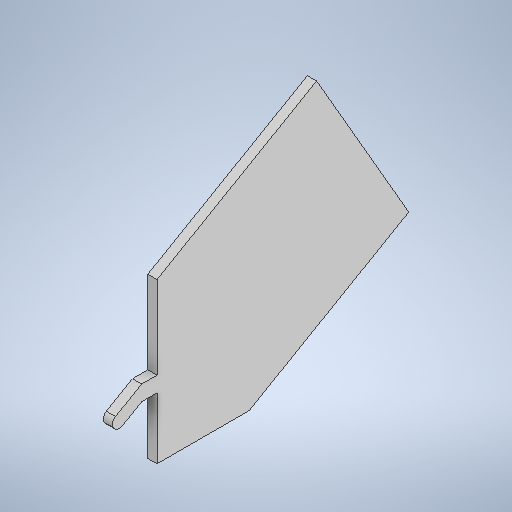
# Autodesk Inventor part: autour hélice
Saved by Autodesk Inventor 2026.2 (Build 302298010, 298A)
## iProperties
Created: 2026-04-02
Part Number: autour hélice
Material: Générique
Document SubType Name: Modeling
Designer: Genon
Density: 1 g/cm^3
Appearance: Par défaut
Author: Genon
Autodesk Inventor part; units mm, degrees
ref_plane "YZ Plane" through (0, 0, 0) normal (1, 0, 0) x (0, 1, 0)
ref_plane "XZ Plane" through (0, 0, 0) normal (0, 1, 0) x (-1, 0, 0)
ref_plane "Plan de construction1" through (0, 0, 0) normal (0, 0.5, -0.8660254) x (1, 0, 0)
sketch "Esquisse1" plane through (0, 0, 0) normal (0, 0.5, -0.8660254) x (1, 0, 0)
  line L0 (-40, 0) -> (-40, -30)
  line L1 (-40, -30) -> (-37, -30)
  line L2 (-40, -30) -> (-37, -30)
  line L3 (-37, -30) -> (-37, 30)
  line L4 (-37, 30) -> (-40, 30)
  line L5 (-40, 30) -> (-40, -30)
  point P0 (0, 0)
  point P1 (-37, 0)
  point P2 (-37, -30)
  dimension "d2" = 30
  dimension "d3" = 3
  dimension "d4" = 60
  dimension "d49" = 37
  dimension "d50" = 40
  constraints: 12 end point, 2 horizontal, 2 midpoint, 2 parallel, 1 perpendicular, 1 vertical
  measures "d2" distance of L0.start L0.end
  measures "d3" distance of L0.end L1.end
  measures "d4" distance of L3.end L2.end
  measures "d49" distance of point (0, 0) point (-37, 0)
  measures "d50" distance of point (0, 0) point (-40, 0)
extrude "Extrusion1" add sketch "Esquisse1" along normal blind 60
ref_plane "Plan de construction2" through (0, 0, 15) normal (0, 0, 1) x (1, 0, 0)
sketch "Esquisse2" plane through (0, 0, 15) normal (0, 0, 1) x (1, 0, 0)
  line L0 (-40, -25.9808) -> (-40, 25.9808) projected
  line L1 (-37, 25.9808) -> (-37, -25.9808) projected
  line L2 (-40, 25.9808) -> (-37, 25.9808) projected
  line L3 (-37, -25.9808) -> (-40, -25.9808) projected
  line L4 (-37, 55.9808) -> (-37, 4.0192) projected
  line L5 (-40, 25.9808) -> (-37, 25.9808)
  line L6 (-37, 25.9808) -> (-37, 35.9808)
  line L7 (-37, 35.9808) -> (-40, 35.9808)
  line L8 (-40, 35.9808) -> (-40, 25.9808)
  point P0 (0, 0)
  point P1 (37, 25.9808)
  dimension "d46" = 10
  constraints: 8 end point, 2 parallel, 1 horizontal, 1 perpendicular, 1 point on line
  measures "d46" distance of L6.end L5.end
extrude "Extrusion2" add sketch "Esquisse2" against normal blind 30 contours L0 L2 L1 L3
ref_plane "Plan de construction3" through (-37, -25.9808, 15) normal (1, 0, 0) x (0, 0, -1)
sketch "Esquisse3" plane through (-37, -25.9808, 15) normal (1, 0, 0) x (0, 0, -1)
  line L0 (0, 0) -> (0, 20)
  line L1 (0, 51.9615) -> (0, 0) projected
  line L2 (0, 20) -> (-5, 20)
  line L3 (-5, 20) -> (-5, 25)
  line L4 (-5, 25) -> (0, 25)
  point P0 (15, 25.9808)
  dimension "d16" = 20
  dimension "d17" = 5
  constraints: 8 end point, 2 perpendicular, 2 point on line, 1 vertical
  measures "d16" distance of L0.start L0.end
  measures "d17" distance of L0.end L2.end
extrude "Extrusion3" add sketch "Esquisse3" against normal up to surface (3 mm away)
ref_plane "Plan de construction6" through (0, -11.0705, 19.1747) normal (0, 0.5, -0.8660254) x (1, 0, 0)
sketch "Esquisse5" plane through (0, -11.0705, 19.1747) normal (0, 0.5, -0.8660254) x (1, 0, 0)
  line L0 (-40, -9.1506) -> (-40, -4.8205) projected
  line L1 (-37, -9.1506) -> (-40, -9.1506) projected
  line L2 (-37, -4.8205) -> (-40, -4.8205) projected
  line L3 (-37, -9.1506) -> (-37, -4.8205) projected
  point P0 (0, 0)
extrude "Extrusion5" add sketch "Esquisse5" along normal mid plane 15
fillet "Congé1" radius 2 2 edges at (-38.5, -6.8958, 30.2452) (-38.5, -10.6458, 28.0801)
sketch "Esquisse12" plane through (-37, -25.9808, 15) normal (1, 0, 0) x (0, 0, -1)
  line L0 (0, 25) -> (-1.3397, 25) projected
  line L1 (0, 25) -> (-6.1432, 25)
  line L2 (-6.1432, 25) -> (-6.1432, 29.4942)
  line L3 (-6.1432, 29.4942) -> (0, 29.4942)
  line L4 (0, 29.4942) -> (0, 25)
  point P0 (15, 25.9808)
  constraints: 8 end point, 2 parallel, 1 horizontal, 1 perpendicular
extrude "Extrusion11" cut sketch "Esquisse12" against normal through all
